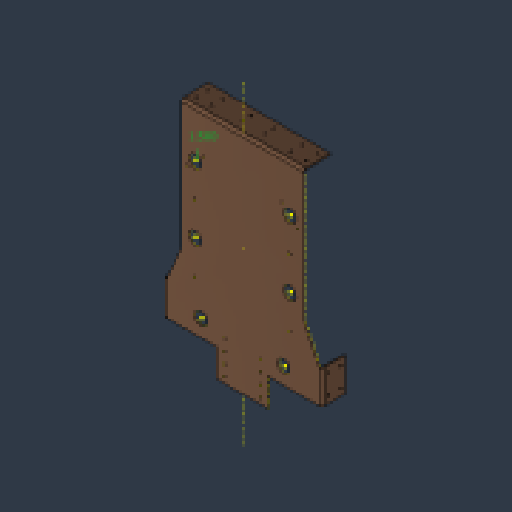
# Autodesk Inventor part: feeder_bottom_plate
Saved by Autodesk Inventor 2024.3 (Build 283343000, 343)
## iProperties
Created: 2025-03-07
Part Number: feeder_bottom_plate
Material: Aluminum 6061
Document SubType Name: Sheet Metal
Designer: marcu
Density: 2.7 g/cm^3
Sheet Metal Rule: Default
Appearance: Aluminum - Flat
Mass: 4544.64 g
Surface Area: 3325.9 cm^2
Volume: 512.361 cm^3
Author: marcu
Autodesk Inventor part; units mm, degrees
ref_plane "YZ Plane" through (0, 0, 0) normal (1, 0, 0) x (0, 1, 0)
ref_plane "XZ Plane" through (0, 0, 0) normal (0, 1, 0) x (-1, 0, 0)
ref_plane "XY Plane" through (0, 0, 0) normal (0, 0, 1) x (1, 0, 0)
sketch "Sketch1" plane through (0, 0, 0) normal (0, 0, 1) x (1, 0, 0)
  line L0 (139.7, -222.25) -> (-139.7, -222.25)
  line L1 (-139.7, -222.25) -> (-139.7, -69.85) construction
  line L2 (-139.7, 222.25) -> (139.7, 222.25)
  line L3 (139.7, 222.25) -> (139.7, -69.85)
  line L4 (139.7, -222.25) -> (-139.7, 222.25) construction
  line L5 (-139.7, -222.25) -> (139.7, 222.25) construction
  line L6 (-139.7, 222.25) -> (-50.8, 222.25)
  line L7 (-139.7, 209.55) -> (-139.7, 222.25)
  line L8 (139.7, 222.25) -> (50.8, 222.25)
  line L9 (139.7, 209.55) -> (139.7, 222.25)
  line L10 (-57.15, -222.25) -> (57.15, -222.25)
  line L11 (57.15, -222.25) -> (57.15, -311.15)
  line L12 (57.15, -311.15) -> (-57.15, -311.15)
  line L13 (-57.15, -311.15) -> (-57.15, -222.25)
  line L14 (0, 328.93) -> (0, -417.83)
  line L15 (-139.7, -222.25) -> (-174.625, -222.25)
  line L16 (-174.625, -222.25) -> (-174.625, -146.05)
  line L17 (-174.625, -146.05) -> (-139.7, -146.05) construction
  line L18 (-139.7, -146.05) -> (-139.7, -222.25) construction
  line L19 (-174.625, -146.05) -> (-139.7, -69.85)
  line L20 (-139.7, -69.85) -> (-139.7, 222.25)
  line L21 (139.7, -146.05) -> (139.7, -222.25)
  line L22 (139.7, -222.25) -> (174.625, -222.25)
  line L23 (174.625, -222.25) -> (174.625, -146.05)
  line L24 (174.625, -146.05) -> (139.7, -146.05) construction
  line L25 (139.7, -146.05) -> (139.7, -222.25)
  line L26 (174.625, -146.05) -> (139.7, -69.85)
  line L27 (139.7, -69.85) -> (139.7, -222.25) construction
  point P0 (0, 0)
  point P1 (0, -311.15)
  dimension "d0" = 279.4
  dimension "d1" = 444.5
  dimension "d76" = 114.3
  dimension "d77" = 88.9
  dimension "d114" = 34.925
  dimension "d115" = 76.2
  dimension "d117" = 152.4
  measures "d0" distance of L2.start L2.end
  measures "d1" distance of L0.end L2.start
  measures "d76" distance of L11.end L12.end
  measures "d77" distance between parallel lines of L0 L12
  measures "d114" distance of L16.end L17.end
  measures "d115" distance of L15.end L16.end
  measures "d117" distance from line of L0 L1.end
extrude "Plate1" add sketch "Sketch1" along normal blind 3.175 contours L0 L14 L2 L3 L26 L23 L22 | L0 L15 L16 L19 L20 L7 L2 L14
sketch "Sketch2" plane through (0, 0, 0) normal (0, 0, -1) x (-1, 0, 0)
  line L0 (107.95, 120.65) -> (-107.95, 120.65) construction
  line L1 (-139.7, 222.25) -> (139.7, 222.25) construction
  line L2 (139.7, -222.25) -> (139.7, 222.25) construction
  line L3 (107.95, -32.004) -> (94.6453, -184.0771) construction
  line L4 (107.95, -32.004) -> (260.604, -32.004) construction
  line L5 (-107.95, -32.004) -> (-94.6453, -184.0771) construction
  line L6 (-107.95, -32.004) -> (44.704, -32.004) construction
  point P0 (0, 0)
  point P1 (0, 120.65)
  point P2 (0, 222.25)
  point P3 (-50.8, 222.25)
  point P4 (50.8, 222.25)
  point P5 (139.7, 209.55)
  dimension "d3" = 215.9
  dimension "d4" = 101.6
  dimension "d14" = 152.654
  dimension "d164" = 152.654
  dimension "d165" = 95
  dimension "d166" = 152.654
  dimension "d167" = 85
  constraints: 10 end point, 4 coincident, 3 horizontal, 2 equal length, 2 midpoint, 1 vertical, 1 vertical alignment, 2 other
  measures "d3" distance of L0.start L0.end
  measures "d4" distance between parallel lines of L0 L1
  measures "d14" distance of point (107.95, 120.65) L3.start
  measures "d164" distance of L3.start L3.end
  measures "d165" angle of L3 L4
  measures "d166" distance of L5.start L5.end
  measures "d167" angle of L5 L6
hole "Hole1" at (-107.95, 120.65, 0) at (107.95, 120.65, 0) at (-107.95, -32.004, 0) at (107.95, -32.004, 0) at (-94.6453, -184.0771, 0) at (94.6453, -184.0771, 0) direction (0, 0, 1) diameter 28.575 end through all
sketch "Sketch3" plane through (139.7, 225.425, -3.175) normal (0, 1, 0) x (-1, 0, 0)
  line L0 (279.4, 0) -> (0, 0)
  line L1 (0, 0) -> (0, -55.5625)
  line L2 (0, -55.5625) -> (279.4, -55.5625)
  line L3 (279.4, -55.5625) -> (279.4, 0)
  constraints: 6 end point, 1 horizontal, 1 perpendicular, 1 vertical
edge flange "Flange1" height 58.7375 angle 90 thickness 3.175 bend radius 3.175 thickness toward (0, 1, 0) relief straight relief width 3.175 relief depth 1.5875 edges at (0, 222.25, 0) wall of the first edge with corners at (-139.7, 225.425, -3.175) (139.7, 225.425, -3.175) (139.7, 225.425, -58.7375) (-139.7, 225.425, -58.7375)
bend "Bend1"
corner "Corner1"
sketch "Sketch4" plane through (-139.7, 228.6, -58.7375) normal (0, 1, 0) x (1, 0, 0)
  line L0 (0, -55.5625) -> (279.4, -55.5625) construction
  line L1 (279.4, 0) -> (279.4, -55.5625) construction
  line L2 (0, 0) -> (279.4, 0) construction
  line L3 (0, -55.5625) -> (0, 0) construction
  point P0 (139.7, -58.7375)
  point P1 (114.3, -34.925)
  point P2 (165.1, -34.925)
  point P3 (114.3, -15.875)
  point P4 (165.1, -15.875)
  dimension "d33" = 114.3
  dimension "d34" = 114.3
  dimension "d37" = 19.05
  dimension "d61" = 15.875
  constraints: 1 horizontal alignment, 1 vertical, 2 other
  measures "d33" distance from line of L3 point (114.3, -34.925)
  measures "d34" distance from line of L1 point (165.1, -34.925)
  measures "d37" distance of point (114.3, -34.925) point (114.3, -15.875)
  measures "d61" distance from line of L2 point (114.3, -15.875)
hole "Hole2" at (-25.4, 228.6, -23.8125) at (25.4, 228.6, -23.8125) at (-25.4, 228.6, -42.8625) at (25.4, 228.6, -42.8625) direction (0, -1, 0) diameter 5.1054 end through all clearance for "Flat Head Machine Screw (82)" size "#10" standard "Ansi Unified Screw Threads"
sketch "Sketch5" plane through (0, 0, 0) normal (0, 0, -1) x (-1, 0, 0)
  circle A0 centre (-107.95, -32.004) radius 14.2875 construction
  circle A1 centre (107.95, -32.004) radius 14.2875 construction
  circle A2 centre (-107.95, 120.65) radius 14.2875 construction
  circle A3 centre (107.95, 120.65) radius 14.2875 construction
  line L0 (-139.7, -69.85) -> (-139.7, 222.25) construction
  line L1 (174.625, -222.25) -> (-174.625, -222.25) construction
  line L2 (-139.7, 222.25) -> (139.7, 222.25) construction
  line L3 (107.95, 120.65) -> (107.95, -32.004) construction
  line L4 (107.95, -32.004) -> (107.95, -184.658) construction
  line L5 (0, 0) -> (0, -25.4) construction
  line L6 (174.625, -146.05) -> (174.625, -222.25) projected
  line L7 (139.7, -69.85) -> (174.625, -146.05) projected
  line L8 (139.7, 222.25) -> (139.7, -69.85) projected
  line L9 (-174.625, -146.05) -> (-139.7, -69.85) projected
  line L10 (-174.625, -222.25) -> (-174.625, -146.05) projected
  point P0 (107.95, -108.331)
  point P1 (107.95, 44.323)
  dimension "d53" = -25.4
  constraints: 6 end point, 2 midpoint, 2 vertical, 1 collinear
  measures "d53" distance of L5.start L5.end
hole "Hole3" at (-107.95, -108.331, 0) at (-107.95, 44.323, 0) direction (0, 0, 1) diameter 5.1054 end through all clearance for "Flat Head Machine Screw (82)" size "#10" standard "Ansi Unified Screw Threads"
sketch "Sketch9" plane through (0, 0, 3.175) normal (0, 0, 1) x (1, 0, 0)
  circle A0 centre (107.95, 120.65) radius 14.2875 projected
  circle A1 centre (107.95, 120.65) radius 25.4 construction
  line L0 (89.9895, 138.6105) -> (125.9105, 102.6895) construction
  line L1 (107.95, 146.05) -> (107.95, 95.25) construction
  point P0 (0, 0)
  point P1 (107.95, 120.65)
  dimension "d85" = 50.8
  dimension "d86" = 45
  constraints: 4 end point, 4 point on circle, 3 coincident, 3 midpoint, 1 centre point, 1 vertical
  measures "d85" diameter of A1
  measures "d86" angle of L0 L1
hole "Hole4" at (89.9895, 138.6105, 3.175) at (125.9105, 102.6895, 3.175) direction (0, 0, -1) diameter 4.0386 end through all
mirror "Mirror1" about plane through (0, 0, 0) normal (1, 0, 0) of "Hole4"
mirror "Mirror2" about plane through (0, 0, 0) normal (1, 0, 0) of "Hole3"
sketch "Sketch12" plane through (0, 0, 0) normal (0, 0, -1) x (-1, 0, 0)
  line L0 (174.625, -222.25) -> (174.625, -222.25)
  line L1 (58.7375, -222.25) -> (-58.7375, -222.25)
  line L2 (-58.7375, -222.25) -> (-58.7375, -285.75)
  line L3 (-58.7375, -285.75) -> (58.7375, -285.75)
  line L4 (58.7375, -285.75) -> (58.7375, -222.25)
  line L5 (0, -387.35) -> (0, 323.85) construction
  point P0 (0, 0)
  point P1 (-139.7, -222.25)
  point P2 (139.7, -222.25)
  point P3 (0, -285.75)
  point P4 (0, -222.25)
  dimension "d107" = 63.5
  dimension "d108" = 117.475
  measures "d108" distance between parallel lines of L2 L4
sheet face with bend "Face3" sketch "Sketch12" thickness 3.175 toward (0, 0, 1) bend radius 3.175 relief straight relief width 3.175 relief depth 1.5875
bend "Bend4"
sketch "Sketch13" plane through (-177.8, -146.05, -3.175) normal (-1, 0, 0) x (0, -1, 0)
  line L0 (76.2, 0) -> (0, 0)
  line L1 (0, 0) -> (0, -49.2125)
  line L2 (0, -49.2125) -> (76.2, -49.2125)
  line L3 (76.2, -49.2125) -> (76.2, 0)
  constraints: 6 end point, 1 horizontal, 1 perpendicular, 1 vertical
edge flange "Flange3" height 55.5625 angle 90 thickness 3.175 bend radius 3.175 thickness toward (-1, 0, 0) relief straight relief width 3.175 relief depth 1.5875 corner gap 3.175 corner form 0 edges at (-174.625, -184.15, 0) (174.625, -184.15, 0) wall of the first edge with corners at (-177.8, -222.25, -3.175) (-177.8, -146.05, -3.175) (-177.8, -146.05, -52.3875) (-177.8, -222.25, -52.3875)
bend "Bend5"
corner "Corner3"
sketch "Sketch14" plane through (-180.975, -222.25, -52.3875) normal (-1, 0, 0) x (0, 0, 1)
  line L0 (49.2125, 0) -> (0, 0) projected
  line L1 (55.5625, 0) -> (55.5625, 76.2) projected
  point P0 (52.3875, 222.25)
  point P1 (11.1125, 15.875)
  point P2 (11.1125, 60.325)
  point P3 (39.6875, 60.325)
  point P4 (39.6875, 15.875)
  dimension "d130" = 15.875
  dimension "d131" = 44.45
  dimension "d132" = 28.575
  dimension "d133" = 15.875
  constraints: 2 horizontal alignment, 2 vertical alignment
  measures "d130" distance from line of L0 point (11.112, 15.875)
  measures "d131" distance of point (11.112, 60.325) point (11.112, 15.875)
  measures "d132" distance of point (11.112, 15.875) point (39.687, 15.875)
  measures "d133" distance from line of L1 point (39.687, 15.875)
hole "Hole6" at (-180.975, -206.375, -41.275) at (-180.975, -161.925, -41.275) at (-180.975, -161.925, -12.7) at (-180.975, -206.375, -12.7) direction (1, 0, 0) diameter 5.1054 end through all
sketch "Sketch15" plane through (-139.7, 228.6, -58.7375) normal (0, 1, 0) x (1, 0, 0)
  line L0 (0, -55.5625) -> (0, 0) projected
  line L1 (0, 0) -> (279.4, 0) projected
  line L2 (0, -61.9125) -> (279.4, -61.9125) projected
  line L3 (0, -55.5625) -> (279.4, -55.5625) projected
  point P0 (139.7, -58.7375)
  point P1 (14.2875, -15.875)
  point P2 (49.2125, -15.875)
  point P3 (49.2125, -41.275)
  point P4 (14.2875, -41.275)
  dimension "d141" = 14.2875
  dimension "d143" = 25.4
  dimension "d144" = 34.925
  dimension "d153" = 14.2875
  constraints: 2 horizontal alignment, 2 vertical alignment
  measures "d141" distance from line of L0 point (14.287, -15.875)
  measures "d143" distance of point (14.287, -41.275) point (14.287, -15.875)
  measures "d144" distance of point (49.212, -15.875) point (14.287, -15.875)
  measures "d153" distance from line of L3 point (14.287, -41.275)
hole "Hole7" at (-125.4125, 228.6, -42.8625) at (-90.4875, 228.6, -42.8625) at (-90.4875, 228.6, -17.4625) at (-125.4125, 228.6, -17.4625) direction (0, -1, 0) diameter 5.1054 end through all
mirror "Mirror3" about plane through (0, 0, 0) normal (1, 0, 0) of "Hole7"
sketch "Sketch16" plane through (0, 0, 3.175) normal (0, 0, 1) x (1, 0, 0)
  line L0 (-41.275, -273.05) -> (-41.275, -171.45) construction
  line L1 (-58.7375, -285.75) -> (-58.7375, -222.25) construction
  line L2 (58.7375, -285.75) -> (-58.7375, -285.75) projected
  line L3 (-41.275, -273.05) -> (-41.275, -222.25) construction
  line L4 (-41.275, -222.25) -> (-41.275, -171.45) construction
  point P0 (0, 0)
  point P1 (-41.275, -196.85)
  point P2 (-41.275, -247.65)
  dimension "d154" = 17.4625
  dimension "d155" = 12.7
  dimension "d156" = 101.6
  constraints: 6 end point, 3 midpoint, 2 coincident, 1 collinear, 1 vertical
  measures "d154" distance between parallel lines of L1 L0
  measures "d155" distance from line of L2 L0.start
  measures "d156" distance of L0.start L0.end
hole "Hole8" at (-41.275, -196.85, 3.175) at (-41.275, -222.25, 3.175) at (-41.275, -247.65, 3.175) at (-41.275, -273.05, 3.175) direction (0, 0, -1) diameter 4.5 depth 3.175 tip angle 118
mirror "Mirror4" about plane through (0, 0, 0) normal (1, 0, 0) of "Hole8"
sketch "Sketch17" plane through (0, 0, 0) normal (0, 0, -1) x (-1, 0, 0)
  circle A0 centre (-41.275, -273.05) radius 2.25 construction
  circle A1 centre (-41.275, -247.65) radius 2.25 construction
  circle A2 centre (-41.275, -222.25) radius 2.25 construction
  circle A3 centre (-41.275, -196.85) radius 2.25 construction
  circle A4 centre (41.275, -273.05) radius 2.25 construction
  circle A5 centre (41.275, -247.65) radius 2.25 construction
  circle A6 centre (41.275, -222.25) radius 2.25 construction
  circle A7 centre (41.275, -196.85) radius 2.25 construction
  circle A8 centre (-107.95, 44.323) radius 2.5527 construction
  circle A9 centre (-107.95, -108.331) radius 2.5527 construction
  circle A10 centre (125.9105, 102.6895) radius 2.0193 construction
  circle A11 centre (89.9895, 138.6105) radius 2.0193 construction
  circle A12 centre (-125.9105, 102.6895) radius 2.0193 construction
  circle A13 centre (-89.9895, 138.6105) radius 2.0193 construction
  circle A14 centre (107.95, 44.323) radius 2.5527 construction
  circle A15 centre (107.95, -108.331) radius 2.5527 construction
  circle A16 centre (-94.6453, -184.0771) radius 14.2875 construction
  circle A17 centre (94.6453, -184.0771) radius 14.2875 construction
  circle A18 centre (-107.95, -32.004) radius 14.2875 construction
  circle A19 centre (107.95, -32.004) radius 14.2875 construction
  circle A20 centre (-107.95, 120.65) radius 14.2875 construction
  circle A21 centre (107.95, 120.65) radius 14.2875 construction
  line L0 (174.625, -222.25) -> (58.7375, -222.25) construction
  line L1 (174.625, -146.05) -> (174.625, -222.25) construction
  line L2 (139.7, -69.85) -> (174.625, -146.05) construction
  line L3 (139.7, 222.25) -> (139.7, -69.85) construction
  line L4 (-139.7, 222.25) -> (139.7, 222.25) construction
  line L5 (-139.7, -69.85) -> (-139.7, 222.25) construction
  line L6 (-174.625, -146.05) -> (-139.7, -69.85) construction
  line L7 (-174.625, -222.25) -> (-174.625, -146.05) construction
  line L8 (-58.7375, -222.25) -> (-174.625, -222.25) construction
  line L9 (-58.7375, -222.25) -> (-58.7375, -285.75) construction
  line L10 (-58.7375, -285.75) -> (58.7375, -285.75) construction
  line L11 (58.7375, -285.75) -> (58.7375, -222.25) construction
  line L12 (69.85, 222.25) -> (69.85, -222.25)
  line L13 (174.625, -222.25) -> (58.7375, -222.25) construction
  line L14 (0, -388.62) -> (0, 331.47) construction
  line L15 (-69.85, 222.25) -> (-69.85, -222.25)
  line L16 (69.85, 222.25) -> (-69.85, 222.25)
  line L17 (69.85, -222.25) -> (-69.85, -222.25)
  line L18 (12.7, -222.25) -> (-12.7, -222.25)
  line L19 (-12.7, -222.25) -> (-12.7, 222.25)
  line L20 (-12.7, 222.25) -> (12.7, 222.25)
  line L21 (12.7, 222.25) -> (12.7, -222.25)
  line L22 (69.85, 222.25) -> (12.7, 165.1) construction
  line L23 (65.3599, 226.7401) -> (8.2099, 169.5901)
  line L24 (17.1901, 160.6099) -> (74.3401, 217.7599)
  arc A22 (74.3401, 217.7599) -> (65.3599, 226.7401) centre (69.85, 222.25) ccw
  arc A23 (8.2099, 169.5901) -> (17.1901, 160.6099) centre (12.7, 165.1) ccw
  line L25 (69.85, 222.25) -> (150.6723, 222.25) construction
  line L26 (12.7, 165.1) -> (69.85, 107.95) construction
  line L27 (8.2099, 160.6099) -> (65.3599, 103.4599)
  line L28 (74.3401, 112.4401) -> (17.1901, 169.5901)
  arc A24 (17.1901, 169.5901) -> (8.2099, 160.6099) centre (12.7, 165.1) ccw
  arc A25 (65.3599, 103.4599) -> (74.3401, 112.4401) centre (69.85, 107.95) ccw
  line L29 (69.85, 107.95) -> (12.7, 50.8) construction
  line L30 (65.3599, 112.4401) -> (8.2099, 55.2901)
  line L31 (17.1901, 46.3099) -> (74.3401, 103.4599)
  arc A26 (74.3401, 103.4599) -> (65.3599, 112.4401) centre (69.85, 107.95) ccw
  arc A27 (8.2099, 55.2901) -> (17.1901, 46.3099) centre (12.7, 50.8) ccw
  line L32 (12.7, 50.8) -> (69.85, -6.35) construction
  line L33 (8.2099, 46.3099) -> (65.3599, -10.8401)
  line L34 (74.3401, -1.8599) -> (17.1901, 55.2901)
  arc A28 (17.1901, 55.2901) -> (8.2099, 46.3099) centre (12.7, 50.8) ccw
  arc A29 (65.3599, -10.8401) -> (74.3401, -1.8599) centre (69.85, -6.35) ccw
  line L35 (69.85, -6.35) -> (12.7, -63.5) construction
  line L36 (65.3599, -1.8599) -> (8.2099, -59.0099)
  line L37 (17.1901, -67.9901) -> (74.3401, -10.8401)
  arc A30 (74.3401, -10.8401) -> (65.3599, -1.8599) centre (69.85, -6.35) ccw
  arc A31 (8.2099, -59.0099) -> (17.1901, -67.9901) centre (12.7, -63.5) ccw
  line L38 (12.7, -63.5) -> (69.85, -120.65) construction
  line L39 (8.2099, -67.9901) -> (65.3599, -125.1401)
  line L40 (74.3401, -116.1599) -> (17.1901, -59.0099)
  arc A32 (17.1901, -59.0099) -> (8.2099, -67.9901) centre (12.7, -63.5) ccw
  arc A33 (65.3599, -125.1401) -> (74.3401, -116.1599) centre (69.85, -120.65) ccw
  line L41 (69.85, -120.65) -> (12.7, -177.8) construction
  line L42 (65.3599, -116.1599) -> (8.2099, -173.3099)
  line L43 (17.1901, -182.2901) -> (74.3401, -125.1401)
  arc A34 (74.3401, -125.1401) -> (65.3599, -116.1599) centre (69.85, -120.65) ccw
  arc A35 (8.2099, -173.3099) -> (17.1901, -182.2901) centre (12.7, -177.8) ccw
  line L44 (12.7, -177.8) -> (69.85, -177.8)
  line L45 (-65.3599, 226.7401) -> (-8.2099, 169.5901)
  line L46 (-17.1901, 160.6099) -> (-74.3401, 217.7599)
  line L47 (-8.2099, 160.6099) -> (-65.3599, 103.4599)
  line L48 (-74.3401, 112.4401) -> (-17.1901, 169.5901)
  line L49 (-65.3599, 112.4401) -> (-8.2099, 55.2901)
  line L50 (-17.1901, 46.3099) -> (-74.3401, 103.4599)
  line L51 (-8.2099, 46.3099) -> (-65.3599, -10.8401)
  line L52 (-74.3401, -1.8599) -> (-17.1901, 55.2901)
  line L53 (-65.3599, -1.8599) -> (-8.2099, -59.0099)
  line L54 (-17.1901, -67.9901) -> (-74.3401, -10.8401)
  line L55 (-8.2099, -67.9901) -> (-65.3599, -125.1401)
  line L56 (-74.3401, -116.1599) -> (-17.1901, -59.0099)
  line L57 (-65.3599, -116.1599) -> (-8.2099, -173.3099)
  line L58 (-17.1901, -182.2901) -> (-74.3401, -125.1401)
  line L59 (-12.7, -177.8) -> (-69.85, -177.8)
  point P0 (0, 0)
  point P1 (0, -222.25)
  point P2 (41.275, 193.675)
  point P3 (41.275, 136.525)
  point P4 (41.275, 79.375)
  point P5 (41.275, 22.225)
  point P6 (41.275, -34.925)
  point P7 (41.275, -92.075)
  point P8 (41.275, -149.225)
  point P9 (-21.6803, -177.8)
  point P10 (-69.85, -129.6303)
  point P11 (21.6803, -177.8)
  point P12 (69.85, -129.6303)
  point P13 (-12.7, -72.4803)
  point P14 (-60.8697, -120.65)
  point P15 (-12.7, -168.8197)
  point P16 (12.7, -168.8197)
  point P17 (60.8697, -120.65)
  point P18 (12.7, -72.4803)
  point P19 (21.6803, -63.5)
  point P20 (69.85, -111.6697)
  point P21 (69.85, -15.3303)
  point P22 (-21.6803, -63.5)
  point P23 (-69.85, -15.3303)
  point P24 (-69.85, -111.6697)
  point P25 (-12.7, 41.8197)
  point P26 (-60.8697, -6.35)
  point P27 (-12.7, -54.5197)
  point P28 (12.7, -54.5197)
  point P29 (60.8697, -6.35)
  point P30 (12.7, 41.8197)
  point P31 (21.6803, 50.8)
  point P32 (69.85, 2.6303)
  point P33 (69.85, 98.9697)
  point P34 (-21.6803, 50.8)
  point P35 (-69.85, 98.9697)
  point P36 (-69.85, 2.6303)
  point P37 (12.7, 59.7803)
  point P38 (60.8697, 107.95)
  point P39 (12.7, 156.1197)
  point P40 (-12.7, 156.1197)
  point P41 (-60.8697, 107.95)
  point P42 (-12.7, 59.7803)
  point P43 (-21.6803, 165.1)
  point P44 (-69.85, 213.2697)
  point P45 (-69.85, 116.9303)
  point P46 (21.6803, 165.1)
  point P47 (69.85, 116.9303)
  point P48 (69.85, 213.2697)
  dimension "d168" = 38.1
  dimension "d169" = 25.4
  dimension "d170" = 135
  dimension "d171" = 12.7
  dimension "d172" = 12.7
  dimension "d173" = 12.7
  dimension "d174" = 12.7
  dimension "d175" = 12.7
  dimension "d176" = 12.7
  dimension "d177" = 12.7
  constraints: 106 end point, 32 symmetric about line, 28 point on circle, 28 tangent, 14 centre point, 13 point on line, 11 perpendicular, 9 midpoint, 9 parallel, 1 equal length, 1 horizontal
  measures "d168" distance from line of A21.centre L12
  measures "d169" distance between parallel lines of L21 L19
  measures "d170" angle of L22 L25
  measures "d171" distance between parallel lines of L23 L24
  measures "d172" diameter of A25
  measures "d173" diameter of A27
  measures "d174" diameter of A29
  measures "d175" diameter of A31
  measures "d176" diameter of A33
  measures "d177" diameter of A35
extrude "Extrusion1" cut sketch "Sketch17" against normal blind 3.175 contours L44 L43 L12 | L21 L39 L42 | L40 L37 L12 | L15 L58 L59 | L57 L55 L19 | L15 L54 L56 | L53 L51 L19 | L21 L33 L36 | L34 L31 L12 | L15 L50 L52 | L49 L47 L19 | L15 L46 L48 | L21 L27 L30 | L28 L24 L12
sketch "Sketch18" plane through (0, 0, 0) normal (0, 0, -1) x (-1, 0, 0)
  line L0 (-362.9369, 222.377) -> (362.9369, 222.377) construction
  line L1 (-101.6, 209.677) -> (101.6, 209.677) construction
  line L2 (-139.7, 222.25) -> (139.7, 222.25) construction
  line L3 (101.6, -142.748) -> (-101.6, -142.748) construction
  point P0 (0, 0)
  point P1 (0, 209.677)
  point P2 (0, 222.25)
  dimension "d181" = 203.2
  dimension "d182" = 12.7
  dimension "d183" = 203.2
  dimension "d184" = 352.425
  constraints: 6 end point, 2 horizontal, 2 midpoint, 2 vertical alignment, 1 parallel, 2 other
  measures "d181" distance of L1.start L1.end
  measures "d182" distance between parallel lines of L0 L1
  measures "d183" distance of L3.start L3.end
  measures "d184" distance of L1.end L3.start
hole "Hole9" at (101.6, 209.677, 0) at (-101.6, 209.677, 0) at (-101.6, -142.748, 0) at (101.6, -142.748, 0) direction (0, 0, 1) diameter 5.1054 end through all clearance for "Flat Head Machine Screw (82)" size "#10" standard "Ansi Unified Screw Threads"
equation "\"d10\" = Thickness"
equation "\"d34\" = d33"
equation "\"d92\" = Thickness"
equation "\"d133\" = d130"
equation "\"d139\" = Thickness"
equation "\"d153\" = d141"
equation "\"d162\" = Thickness"
equation "\"d190\" = Thickness"
equation "\"d2\" = Thickness"
equation "\"d22\" = BendReliefWidth"
equation "\"d23\" = BendReliefDepth"
equation "\"d24\" = MinimumRemnant"
equation "\"d25\" = TransitionRadius"
equation "\"d28\" = BendRadius"
equation "\"d29\" = CornerReliefSize"
equation "\"d30\" = GapSize"
equation "\"d31\" = JacobiRadiusSize"
equation "\"d109\" = BendRadius"
equation "\"d110\" = BendReliefWidth"
equation "\"d112\" = MinimumRemnant"
equation "\"d111\" = BendReliefDepth"
equation "\"d113\" = TransitionRadius"
equation "\"d118\" = BendReliefWidth"
equation "\"d119\" = BendReliefDepth"
equation "\"d120\" = MinimumRemnant"
equation "\"d121\" = TransitionRadius"
equation "\"d124\" = BendRadius"
equation "\"d125\" = CornerReliefSize"
equation "\"d126\" = GapSize"
equation "\"d127\" = JacobiRadiusSize"
equation "\"BendRadius\" = Thickness"
equation "\"BendReliefWidth\" = Thickness"
equation "\"BendReliefDepth\" = 0.5 * Thickness"
equation "\"CornerReliefSize\" = 4 * Thickness"
equation "\"MinimumRemnant\" = 2 * Thickness"
equation "\"TransitionRadius\" = BendRadius"
equation "\"JacobiRadiusSize\" = BendRadius"
equation "\"GapSize\" = Thickness"
equation "\"Thickness\" = 3.175"
body "Solid1"
